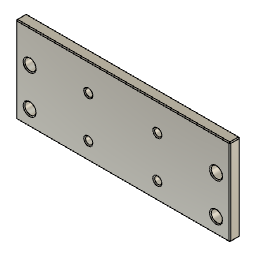
Spindle mount plate (Autodesk Fusion 360 design; units mm, degrees)
Autodesk Fusion 360 part; units mm, degrees
sketch "Plate" plane through (0, 0, 0) normal (0, 1, 0) x (1, 0, 0)
  line L0 (-54, 41.5) -> (54, 41.5) construction
  circle A0 centre (-54, 41.5) radius 3.25
  circle A1 centre (-20, 62.5) radius 2.1
  circle A2 centre (-54, 63.5) radius 3.25
  circle A3 centre (-20, 38.5) radius 2.1
  line L1 (20, 62.5) -> (-20, 62.5) construction
  line L2 (-20, 38.5) -> (20, 38.5) construction
  line L3 (-20, 62.5) -> (-20, 38.5) construction
  line L4 (54, 41.5) -> (54, 63.5) construction
  line L5 (20, 38.5) -> (20, 62.5) construction
  line L6 (54, 63.5) -> (-54, 63.5) construction
  circle A4 centre (54, 63.5) radius 3.25
  circle A5 centre (20, 38.5) radius 2.1
  circle A6 centre (20, 62.5) radius 2.1
  circle A7 centre (54, 41.5) radius 3.25
  line L7 (-54, 63.5) -> (-54, 41.5) construction
  line L8 (-62, 22.5) -> (62, 22.5)
  line L9 (62, 22.5) -> (62, 72.5)
  line L10 (62, 72.5) -> (-62, 72.5)
  line L11 (-62, 72.5) -> (-62, 22.5)
  point P0 (-54.1427, 52.5)
  dimension "d1" = 108
  dimension "d2" = 22
  dimension "d3" = 6.5
  dimension "d4" = 6.5
  dimension "d5" = 6.5
  dimension "d6" = 6.5
  dimension "d7" = 40
  dimension "d8" = 24
  dimension "d9" = 3
  dimension "d10" = 4.2
  dimension "d11" = 4.2
  dimension "d12" = 4.2
  dimension "d13" = 4.2
  dimension "d14" = 124
  dimension "d15" = 50
  dimension "d16" = 8
  dimension "d17" = 7.5
  dimension "d18" = 10
  constraint horizontal L0
  constraint vertical L4
  constraint horizontal L6
  constraint vertical L7
  constraint coincident L0.start A0.centre
  constraint coincident A2.centre L6.end
  constraint coincident L0.end L4.start
  constraint coincident L4.end L6.start
  constraint horizontal L2
  constraint vertical L5
  constraint horizontal L1
  constraint vertical L3
  constraint coincident A3.centre L2.start
  constraint coincident L2.end L5.start
  constraint coincident A1.centre L1.end
  constraint coincident L1.start L5.end
  constraint horizontal L8
  constraint vertical L9
  constraint horizontal L10
  constraint vertical L11
  measures "d1" distance of L0.start L0.end
  measures "d2" distance of A2.centre L0.start
  measures "d3" diameter of A0
  measures "d4" diameter of A2
  measures "d5" diameter of A7
  measures "d6" diameter of A4
  measures "d7" distance of A3.centre L2.end
  measures "d8" distance of A1.centre A3.centre
  measures "d9" distance of L0 L2
  measures "d10" diameter of A3
  measures "d11" diameter of A5
  measures "d12" diameter of A1
  measures "d13" diameter of A6 L10
  measures "d14" distance of L8.start L8.end
  measures "d15" distance of L8.start L10.end
  measures "d16" distance of L0.start L11
  measures "d18" distance of A1.centre L10
extrude "Extrude1" add sketch "Plate" along normal blind 6 makes body 1
copy_body "Body->Comp1" bodies 1 removing the originals makes body 2 in component "Plate"
chamfer "Chamfer1" distance 0.5 angle 45 28 edges at (-62, 0, -47.5) (-62, 3, -22.5) (0, 0, -22.5) (0, 6, -22.5) (62, 3, -22.5) (62, 0, -47.5) (62, 6, -47.5) (0, 0, -72.5) (62, 3, -72.5) (0, 6, -72.5) (-62, 6, -47.5) (-62, 3, -72.5) (-57.0301, 6, -64.6753) (-57.0301, 6, -42.6753) (-21.9579, 6, -39.2594) (-21.9579, 6, -63.2594) (18.0421, 6, -39.2594) (18.0421, 6, -63.2594) (50.9699, 6, -42.6753) (50.9699, 6, -64.6753) (-57.0301, 0, -64.6753) (-57.0301, 0, -42.6753) (-21.9579, 0, -39.2594) (-21.9579, 0, -63.2594) (18.0421, 0, -39.2594) (18.0421, 0, -63.2594) (50.9699, 0, -42.6753) (50.9699, 0, -64.6753) on bodies 2 in component "Plate"
component "Plate" placed x (1, 0, 0) y (0, 1, 0) z (0, 0, 1) at (0, 0, 0)
named bodies: "Plate"
